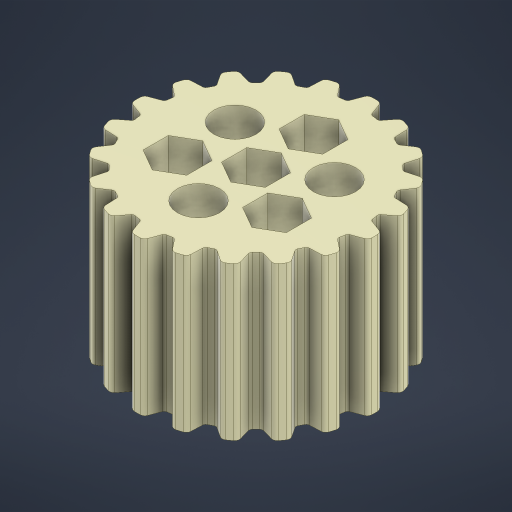
# Autodesk Inventor part: Pulley_Joint2
Saved by Autodesk Inventor 2023 (Build 270158000, 158)
## iProperties
Created: 2023-02-17
Part Number: Pulley_Joint2
Material: ABS Plastic
Document SubType Name: Modeling
Designer: dzw04
Density: 1.06 g/cm^3
Appearance: Smooth - Ash
Author: dzw04
Autodesk Inventor part; units mm, degrees
ref_plane "YZ Plane" through (0, 0, 0) normal (1, 0, 0) x (0, 1, 0)
ref_plane "XZ Plane" through (0, 0, 0) normal (0, 1, 0) x (-1, 0, 0)
ref_plane "XY Plane" through (0, 0, 0) normal (0, 0, 1) x (1, 0, 0)
sketch "Sketch1" plane through (0, 0, 0) normal (0, 1, 0) x (-1, 0, 0)
  arc A0 (-1.7917, 13.431) -> (-2.4464, 13.3273) centre (0, 0) ccw
  arc A1 (-2.8316, 13.4718) -> (-2.4464, 13.3273) centre (-2.5186, 13.7208) ccw
  line L0 (-2.8316, 13.4718) -> (-3.774, 14.6565)
  arc A2 (-3.774, 14.6565) -> (-4.4144, 14.8581) centre (-4.2435, 14.2829) ccw
  arc A3 (-4.4144, 14.8581) -> (-5.162, 14.6152) centre (0, 0) ccw
  arc A4 (-5.162, 14.6152) -> (-5.5616, 14.0756) centre (-4.9622, 14.0494) ccw
  line L1 (-5.5616, 14.0756) -> (-5.6277, 12.5633)
  arc A5 (-5.8545, 12.22) -> (-5.6277, 12.5633) centre (-6.0273, 12.5807) ccw
  arc A6 (-5.8545, 12.22) -> (-6.445, 11.9191) centre (0, 0) ccw
  arc A7 (-6.856, 11.9374) -> (-6.445, 11.9191) centre (-6.6353, 12.2709) ccw
  line L2 (-6.856, 11.9374) -> (-8.1183, 12.7729)
  arc A8 (-8.1183, 12.7729) -> (-8.7898, 12.7668) centre (-8.4495, 12.2726) ccw
  arc A9 (-8.7898, 12.7668) -> (-9.4257, 12.3047) centre (0, 0) ccw
  arc A10 (-9.4257, 12.3047) -> (-9.639, 11.668) centre (-9.0609, 11.8284) ccw
  line L3 (-9.639, 11.668) -> (-9.2345, 10.2093)
  arc A11 (-9.3441, 9.8128) -> (-9.2345, 10.2093) centre (-9.6199, 10.1024) ccw
  arc A12 (-9.3441, 9.8128) -> (-9.8128, 9.3441) centre (0, 0) ccw
  arc A13 (-10.2093, 9.2345) -> (-9.8128, 9.3441) centre (-10.1024, 9.6199) ccw
  line L4 (-10.2093, 9.2345) -> (-11.668, 9.639)
  arc A14 (-11.668, 9.639) -> (-12.3047, 9.4257) centre (-11.8284, 9.0609) ccw
  arc A15 (-12.3047, 9.4257) -> (-12.7668, 8.7898) centre (0, 0) ccw
  arc A16 (-12.7668, 8.7898) -> (-12.7729, 8.1183) centre (-12.2726, 8.4495) ccw
  line L5 (-12.7729, 8.1183) -> (-11.9374, 6.856)
  arc A17 (-11.9191, 6.445) -> (-11.9374, 6.856) centre (-12.2709, 6.6353) ccw
  arc A18 (-11.9191, 6.445) -> (-12.22, 5.8545) centre (0, 0) ccw
  arc A19 (-12.5633, 5.6277) -> (-12.22, 5.8545) centre (-12.5807, 6.0273) ccw
  line L6 (-12.5633, 5.6277) -> (-14.0756, 5.5616)
  arc A20 (-14.0756, 5.5616) -> (-14.6152, 5.162) centre (-14.0494, 4.9622) ccw
  arc A21 (-14.6152, 5.162) -> (-14.8581, 4.4144) centre (0, 0) ccw
  arc A22 (-14.8581, 4.4144) -> (-14.6565, 3.774) centre (-14.2829, 4.2435) ccw
  line L7 (-14.6565, 3.774) -> (-13.4718, 2.8316)
  arc A23 (-13.3273, 2.4464) -> (-13.4718, 2.8316) centre (-13.7208, 2.5186) ccw
  arc A24 (-13.3273, 2.4464) -> (-13.431, 1.7917) centre (0, 0) ccw
  arc A25 (-13.6874, 1.47) -> (-13.431, 1.7917) centre (-13.8275, 1.8446) ccw
  line L8 (-13.6874, 1.47) -> (-15.1053, 0.9398)
  arc A26 (-15.1053, 0.9398) -> (-15.495, 0.393) centre (-14.8952, 0.3778) ccw
  arc A27 (-15.495, 0.393) -> (-15.495, -0.393) centre (0, 0) ccw
  arc A28 (-15.495, -0.393) -> (-15.1053, -0.9398) centre (-14.8952, -0.3778) ccw
  line L9 (-15.1053, -0.9398) -> (-13.6874, -1.47)
  arc A29 (-13.431, -1.7917) -> (-13.6874, -1.47) centre (-13.8275, -1.8446) ccw
  arc A30 (-13.431, -1.7917) -> (-13.3273, -2.4464) centre (0, 0) ccw
  arc A31 (-13.4718, -2.8316) -> (-13.3273, -2.4464) centre (-13.7208, -2.5186) ccw
  line L10 (-13.4718, -2.8316) -> (-14.6565, -3.774)
  arc A32 (-14.6565, -3.774) -> (-14.8581, -4.4144) centre (-14.2829, -4.2435) ccw
  arc A33 (-14.8581, -4.4144) -> (-14.6152, -5.162) centre (0, 0) ccw
  arc A34 (-14.6152, -5.162) -> (-14.0756, -5.5616) centre (-14.0494, -4.9622) ccw
  line L11 (-14.0756, -5.5616) -> (-12.5633, -5.6277)
  arc A35 (-12.22, -5.8545) -> (-12.5633, -5.6277) centre (-12.5807, -6.0273) ccw
  arc A36 (-12.22, -5.8545) -> (-11.9191, -6.445) centre (0, 0) ccw
  arc A37 (-11.9374, -6.856) -> (-11.9191, -6.445) centre (-12.2709, -6.6353) ccw
  line L12 (-11.9374, -6.856) -> (-12.7729, -8.1183)
  arc A38 (-12.7729, -8.1183) -> (-12.7668, -8.7898) centre (-12.2726, -8.4495) ccw
  arc A39 (-12.7668, -8.7898) -> (-12.3047, -9.4257) centre (0, 0) ccw
  arc A40 (-12.3047, -9.4257) -> (-11.668, -9.639) centre (-11.8284, -9.0609) ccw
  line L13 (-11.668, -9.639) -> (-10.2093, -9.2345)
  arc A41 (-9.8128, -9.3441) -> (-10.2093, -9.2345) centre (-10.1024, -9.6199) ccw
  arc A42 (-9.8128, -9.3441) -> (-9.3441, -9.8128) centre (0, 0) ccw
  arc A43 (-9.2345, -10.2093) -> (-9.3441, -9.8128) centre (-9.6199, -10.1024) ccw
  line L14 (-9.2345, -10.2093) -> (-9.639, -11.668)
  arc A44 (-9.639, -11.668) -> (-9.4257, -12.3047) centre (-9.0609, -11.8284) ccw
  arc A45 (-9.4257, -12.3047) -> (-8.7898, -12.7668) centre (0, 0) ccw
  arc A46 (-8.7898, -12.7668) -> (-8.1183, -12.7729) centre (-8.4495, -12.2726) ccw
  line L15 (-8.1183, -12.7729) -> (-6.856, -11.9374)
  arc A47 (-6.445, -11.9191) -> (-6.856, -11.9374) centre (-6.6353, -12.2709) ccw
  arc A48 (-6.445, -11.9191) -> (-5.8545, -12.22) centre (0, 0) ccw
  arc A49 (-5.6277, -12.5633) -> (-5.8545, -12.22) centre (-6.0273, -12.5807) ccw
  line L16 (-5.6277, -12.5633) -> (-5.5616, -14.0756)
  arc A50 (-5.5616, -14.0756) -> (-5.162, -14.6152) centre (-4.9622, -14.0494) ccw
  arc A51 (-5.162, -14.6152) -> (-4.4144, -14.8581) centre (0, 0) ccw
  arc A52 (-4.4144, -14.8581) -> (-3.774, -14.6565) centre (-4.2435, -14.2829) ccw
  line L17 (-3.774, -14.6565) -> (-2.8316, -13.4718)
  arc A53 (-2.4464, -13.3273) -> (-2.8316, -13.4718) centre (-2.5186, -13.7208) ccw
  arc A54 (-2.4464, -13.3273) -> (-1.7917, -13.431) centre (0, 0) ccw
  arc A55 (-1.47, -13.6874) -> (-1.7917, -13.431) centre (-1.8446, -13.8275) ccw
  line L18 (-1.47, -13.6874) -> (-0.9398, -15.1053)
  arc A56 (-0.9398, -15.1053) -> (-0.393, -15.495) centre (-0.3778, -14.8952) ccw
  arc A57 (-0.393, -15.495) -> (0.393, -15.495) centre (0, 0) ccw
  arc A58 (0.393, -15.495) -> (0.9398, -15.1053) centre (0.3778, -14.8952) ccw
  line L19 (0.9398, -15.1053) -> (1.47, -13.6874)
  arc A59 (1.7917, -13.431) -> (1.47, -13.6874) centre (1.8446, -13.8275) ccw
  arc A60 (1.7917, -13.431) -> (2.4464, -13.3273) centre (0, 0) ccw
  arc A61 (2.8316, -13.4718) -> (2.4464, -13.3273) centre (2.5186, -13.7208) ccw
  line L20 (2.8316, -13.4718) -> (3.774, -14.6565)
  arc A62 (3.774, -14.6565) -> (4.4144, -14.8581) centre (4.2435, -14.2829) ccw
  arc A63 (4.4144, -14.8581) -> (5.162, -14.6152) centre (0, 0) ccw
  arc A64 (5.162, -14.6152) -> (5.5616, -14.0756) centre (4.9622, -14.0494) ccw
  line L21 (5.5616, -14.0756) -> (5.6277, -12.5633)
  arc A65 (5.8545, -12.22) -> (5.6277, -12.5633) centre (6.0273, -12.5807) ccw
  arc A66 (5.8545, -12.22) -> (6.445, -11.9191) centre (0, 0) ccw
  arc A67 (6.856, -11.9374) -> (6.445, -11.9191) centre (6.6353, -12.2709) ccw
  line L22 (6.856, -11.9374) -> (8.1183, -12.7729)
  arc A68 (8.1183, -12.7729) -> (8.7898, -12.7668) centre (8.4495, -12.2726) ccw
  arc A69 (8.7898, -12.7668) -> (9.4257, -12.3047) centre (0, 0) ccw
  arc A70 (9.4257, -12.3047) -> (9.639, -11.668) centre (9.0609, -11.8284) ccw
  line L23 (9.639, -11.668) -> (9.2345, -10.2093)
  arc A71 (9.3441, -9.8128) -> (9.2345, -10.2093) centre (9.6199, -10.1024) ccw
  arc A72 (9.3441, -9.8128) -> (9.8128, -9.3441) centre (0, 0) ccw
  arc A73 (10.2093, -9.2345) -> (9.8128, -9.3441) centre (10.1024, -9.6199) ccw
  line L24 (10.2093, -9.2345) -> (11.668, -9.639)
  arc A74 (11.668, -9.639) -> (12.3047, -9.4257) centre (11.8284, -9.0609) ccw
  arc A75 (12.3047, -9.4257) -> (12.7668, -8.7898) centre (0, 0) ccw
  arc A76 (12.7668, -8.7898) -> (12.7729, -8.1183) centre (12.2726, -8.4495) ccw
  line L25 (12.7729, -8.1183) -> (11.9374, -6.856)
  arc A77 (11.9191, -6.445) -> (11.9374, -6.856) centre (12.2709, -6.6353) ccw
  arc A78 (11.9191, -6.445) -> (12.22, -5.8545) centre (0, 0) ccw
  arc A79 (12.5633, -5.6277) -> (12.22, -5.8545) centre (12.5807, -6.0273) ccw
  line L26 (12.5633, -5.6277) -> (14.0756, -5.5616)
  arc A80 (14.0756, -5.5616) -> (14.6152, -5.162) centre (14.0494, -4.9622) ccw
  arc A81 (14.6152, -5.162) -> (14.8581, -4.4144) centre (0, 0) ccw
  arc A82 (14.8581, -4.4144) -> (14.6565, -3.774) centre (14.2829, -4.2435) ccw
  line L27 (14.6565, -3.774) -> (13.4718, -2.8316)
  arc A83 (13.3273, -2.4464) -> (13.4718, -2.8316) centre (13.7208, -2.5186) ccw
  arc A84 (13.3273, -2.4464) -> (13.431, -1.7917) centre (0, 0) ccw
  arc A85 (13.6874, -1.47) -> (13.431, -1.7917) centre (13.8275, -1.8446) ccw
  line L28 (13.6874, -1.47) -> (15.1053, -0.9398)
  arc A86 (15.1053, -0.9398) -> (15.495, -0.393) centre (14.8952, -0.3778) ccw
  arc A87 (15.495, -0.393) -> (15.495, 0.393) centre (0, 0) ccw
  arc A88 (15.495, 0.393) -> (15.1053, 0.9398) centre (14.8952, 0.3778) ccw
  line L29 (15.1053, 0.9398) -> (13.6874, 1.47)
  arc A89 (13.431, 1.7917) -> (13.6874, 1.47) centre (13.8275, 1.8446) ccw
  arc A90 (13.431, 1.7917) -> (13.3273, 2.4464) centre (0, 0) ccw
  arc A91 (13.4718, 2.8316) -> (13.3273, 2.4464) centre (13.7208, 2.5186) ccw
  line L30 (13.4718, 2.8316) -> (14.6565, 3.774)
  arc A92 (14.6565, 3.774) -> (14.8581, 4.4144) centre (14.2829, 4.2435) ccw
  arc A93 (14.8581, 4.4144) -> (14.6152, 5.162) centre (0, 0) ccw
  arc A94 (14.6152, 5.162) -> (14.0756, 5.5616) centre (14.0494, 4.9622) ccw
  line L31 (14.0756, 5.5616) -> (12.5633, 5.6277)
  arc A95 (12.22, 5.8545) -> (12.5633, 5.6277) centre (12.5807, 6.0273) ccw
  arc A96 (12.22, 5.8545) -> (11.9191, 6.445) centre (0, 0) ccw
  arc A97 (11.9374, 6.856) -> (11.9191, 6.445) centre (12.2709, 6.6353) ccw
  line L32 (11.9374, 6.856) -> (12.7729, 8.1183)
  arc A98 (12.7729, 8.1183) -> (12.7668, 8.7898) centre (12.2726, 8.4495) ccw
  arc A99 (12.7668, 8.7898) -> (12.3047, 9.4257) centre (0, 0) ccw
  arc A100 (12.3047, 9.4257) -> (11.668, 9.639) centre (11.8284, 9.0609) ccw
  line L33 (11.668, 9.639) -> (10.2093, 9.2345)
  arc A101 (9.8128, 9.3441) -> (10.2093, 9.2345) centre (10.1024, 9.6199) ccw
  arc A102 (9.8128, 9.3441) -> (9.3441, 9.8128) centre (0, 0) ccw
  arc A103 (9.2345, 10.2093) -> (9.3441, 9.8128) centre (9.6199, 10.1024) ccw
  line L34 (9.2345, 10.2093) -> (9.639, 11.668)
  arc A104 (9.639, 11.668) -> (9.4257, 12.3047) centre (9.0609, 11.8284) ccw
  arc A105 (9.4257, 12.3047) -> (8.7898, 12.7668) centre (0, 0) ccw
  arc A106 (8.7898, 12.7668) -> (8.1183, 12.7729) centre (8.4495, 12.2726) ccw
  line L35 (8.1183, 12.7729) -> (6.856, 11.9374)
  arc A107 (6.445, 11.9191) -> (6.856, 11.9374) centre (6.6353, 12.2709) ccw
  arc A108 (6.445, 11.9191) -> (5.8545, 12.22) centre (0, 0) ccw
  arc A109 (5.6277, 12.5633) -> (5.8545, 12.22) centre (6.0273, 12.5807) ccw
  line L36 (5.6277, 12.5633) -> (5.5616, 14.0756)
  arc A110 (5.5616, 14.0756) -> (5.162, 14.6152) centre (4.9622, 14.0494) ccw
  arc A111 (5.162, 14.6152) -> (4.4144, 14.8581) centre (0, 0) ccw
  arc A112 (4.4144, 14.8581) -> (3.774, 14.6565) centre (4.2435, 14.2829) ccw
  line L37 (3.774, 14.6565) -> (2.8316, 13.4718)
  arc A113 (2.4464, 13.3273) -> (2.8316, 13.4718) centre (2.5186, 13.7208) ccw
  arc A114 (2.4464, 13.3273) -> (1.7917, 13.431) centre (0, 0) ccw
  arc A115 (1.47, 13.6874) -> (1.7917, 13.431) centre (1.8446, 13.8275) ccw
  line L38 (1.47, 13.6874) -> (0.9398, 15.1053)
  arc A116 (0.9398, 15.1053) -> (0.393, 15.495) centre (0.3778, 14.8952) ccw
  arc A117 (0.393, 15.495) -> (-0.393, 15.495) centre (0, 0) ccw
  arc A118 (-0.393, 15.495) -> (-0.9398, 15.1053) centre (-0.3778, 14.8952) ccw
  line L39 (-0.9398, 15.1053) -> (-1.47, 13.6874)
  arc A119 (-1.7917, 13.431) -> (-1.47, 13.6874) centre (-1.8446, 13.8275) ccw
  circle A120 centre (0, 0) radius 17.75
  point P0 (1.47, 13.6874)
  point P1 (0.393, 15.495)
  point P2 (-0.393, 15.495)
  point P3 (-0.9398, 15.1053)
  point P4 (-1.7917, 13.431)
  point P5 (-2.4464, 13.3273)
  point P6 (-2.8316, 13.4718)
  point P7 (-4.4144, 14.8581)
  point P8 (-5.162, 14.6152)
  point P9 (-5.5616, 14.0756)
  point P10 (-5.8545, 12.22)
  point P11 (-6.445, 11.9191)
  point P12 (-8.7898, 12.7668)
  point P13 (-9.4257, 12.3047)
  point P14 (-9.639, 11.668)
  point P15 (-9.3441, 9.8128)
  point P16 (-9.8128, 9.3441)
  point P17 (-10.2093, 9.2345)
  point P18 (-12.3047, 9.4257)
  point P19 (-12.7668, 8.7898)
  point P20 (-11.9191, 6.445)
  point P21 (-12.22, 5.8545)
  point P22 (-12.5633, 5.6277)
  point P23 (-14.6152, 5.162)
  point P24 (-14.8581, 4.4144)
  point P25 (-14.6565, 3.774)
  point P26 (-13.3273, 2.4464)
  point P27 (-13.431, 1.7917)
  point P28 (-13.6874, 1.47)
  point P29 (-15.495, 0.393)
  point P30 (-15.495, -0.393)
  point P31 (-15.1053, -0.9398)
  point P32 (-13.3273, -2.4464)
  point P33 (-13.4718, -2.8316)
  point P34 (-14.8581, -4.4144)
  point P35 (-14.6152, -5.162)
  point P36 (-12.22, -5.8545)
  point P37 (-11.9191, -6.445)
  point P38 (-11.9374, -6.856)
  point P39 (-12.7668, -8.7898)
  point P40 (-12.3047, -9.4257)
  point P41 (-9.8128, -9.3441)
  point P42 (-9.3441, -9.8128)
  point P43 (-9.4257, -12.3047)
  point P44 (-8.7898, -12.7668)
  point P45 (-6.445, -11.9191)
  point P46 (-5.8545, -12.22)
  point P47 (-5.6277, -12.5633)
  point P48 (-5.162, -14.6152)
  point P49 (-4.4144, -14.8581)
  point P50 (-2.4464, -13.3273)
  point P51 (-1.7917, -13.431)
  point P52 (-0.393, -15.495)
  point P53 (0.393, -15.495)
  point P54 (0.9398, -15.1053)
  point P55 (1.7917, -13.431)
  point P56 (2.4464, -13.3273)
  point P57 (2.8316, -13.4718)
  point P58 (4.4144, -14.8581)
  point P59 (5.162, -14.6152)
  point P60 (5.8545, -12.22)
  point P61 (6.445, -11.9191)
  point P62 (8.7898, -12.7668)
  point P63 (9.4257, -12.3047)
  point P64 (9.3441, -9.8128)
  point P65 (9.8128, -9.3441)
  point P66 (10.2093, -9.2345)
  point P67 (12.3047, -9.4257)
  point P68 (12.7668, -8.7898)
  point P69 (12.7729, -8.1183)
  point P70 (12.22, -5.8545)
  point P71 (12.5633, -5.6277)
  point P72 (14.6152, -5.162)
  point P73 (14.8581, -4.4144)
  point P74 (14.6565, -3.774)
  point P75 (13.3273, -2.4464)
  point P76 (13.431, -1.7917)
  point P77 (13.6874, -1.47)
  point P78 (15.495, -0.393)
  point P79 (15.495, 0.393)
  point P80 (15.1053, 0.9398)
  point P81 (13.431, 1.7917)
  point P82 (13.3273, 2.4464)
  point P83 (13.4718, 2.8316)
  point P84 (14.8581, 4.4144)
  point P85 (14.6152, 5.162)
  point P86 (14.0756, 5.5616)
  point P87 (12.22, 5.8545)
  point P88 (11.9191, 6.445)
  point P89 (11.9374, 6.856)
  point P90 (12.7668, 8.7898)
  point P91 (12.3047, 9.4257)
  point P92 (11.668, 9.639)
  point P93 (9.8128, 9.3441)
  point P94 (9.3441, 9.8128)
  point P95 (9.4257, 12.3047)
  point P96 (8.7898, 12.7668)
  point P97 (8.1183, 12.7729)
  point P98 (6.445, 11.9191)
  point P99 (5.8545, 12.22)
  point P100 (5.6277, 12.5633)
  point P101 (5.162, 14.6152)
  point P102 (4.4144, 14.8581)
  point P103 (2.4464, 13.3273)
  point P104 (1.7917, 13.431)
  constraints: 240 point on circle, 121 centre point, 80 end point
extrude "Extrusion1" add sketch "Sketch1" along normal blind 20 contours A119 L39 A118 A117 A116 L38 A115 A114 A113 L37 A112 A111 A110 L36 A109 A108 A107 L35 A106 A105 A104 L34 A103 A102 A101 L33 A100 A99 A98 L32 A97 A96 A95 L31 A94 A93 A92 L30 A91 A90 A89 L29 A88 A87 A86 L28 A85 A84 A83 L27 A82 A81 A80 L26 A79 A78 A77 L25 A76 A75 A74 L24 A73 A72 A71 L23 A70 A69 A68 L22 A67 A66 A65 L21 A64 A63 A62 L20 A61 A60 A59 L19 A58 A57 A56 L18 A55 A54 A53 L17 A52 A51 A50 L16 A49 A48 A47 L15 A46 A45 A44 L14 A43 A42 A41 L13 A40 A39 A38 L12 A37 A36 A35 L11 A34 A33 A32 L10 A31 A30 A29 L9 A28 A27 A26 L8 A25 A24 A23 L7 A22 A21 A20 L6 A19 A18 A17 L5 A16 A15 A14 L4 A13 A12 A11 L3 A10 A9 A8 L2 A7 A6 A5 L1 A4 A3 A2 L0 A1 A0
sketch "Sketch2" plane through (0, 20, 0) normal (0, 1, 0) x (1, 0, 0)
  circle A0 centre (0, 0) radius 7.5 construction
  line L0 (0, 4.2091) -> (-2.85, 5.8546)
  line L1 (-2.85, 5.8546) -> (-2.85, 9.1454)
  line L2 (-2.85, 9.1454) -> (0, 10.7909)
  line L3 (0, 10.7909) -> (2.85, 9.1454)
  line L4 (2.85, 9.1454) -> (2.85, 5.8546)
  line L5 (2.85, 5.8546) -> (0, 4.2091)
  line L6 (0, 3.2909) -> (2.85, 1.6454)
  line L7 (2.85, 1.6454) -> (2.85, -1.6454)
  line L8 (2.85, -1.6454) -> (0, -3.2909)
  line L9 (0, -3.2909) -> (-2.85, -1.6454)
  line L10 (-2.85, -1.6454) -> (-2.85, 1.6454)
  line L11 (-2.85, 1.6454) -> (0, 3.2909)
  circle A1 centre (0, 0) radius 7.5 construction
  line L12 (-3.6452, -2.1046) -> (-3.6452, -5.3954)
  line L13 (-3.6452, -5.3954) -> (-6.4952, -7.0409)
  line L14 (-6.4952, -7.0409) -> (-9.3452, -5.3954)
  line L15 (-9.3452, -5.3954) -> (-9.3452, -2.1046)
  line L16 (-9.3452, -2.1046) -> (-6.4952, -0.4591)
  line L17 (-6.4952, -0.4591) -> (-3.6452, -2.1046)
  circle A2 centre (0, 0) radius 7.5 construction
  line L18 (3.6452, -2.1046) -> (6.4952, -0.4591)
  line L19 (6.4952, -0.4591) -> (9.3452, -2.1046)
  line L20 (9.3452, -2.1046) -> (9.3452, -5.3954)
  line L21 (9.3452, -5.3954) -> (6.4952, -7.0409)
  line L22 (6.4952, -7.0409) -> (3.6452, -5.3954)
  line L23 (3.6452, -5.3954) -> (3.6452, -2.1046)
  point P0 (0, 7.5)
  point P1 (-6.4952, -3.75)
  point P2 (6.4952, -3.75)
  dimension "d2" = 15
  dimension "d3" = 5.7
  dimension "d4" = 5.7
  dimension "d7" = 360
  constraints: 48 end point, 2 coincident, 1 vertical alignment, 80 other
  measures "d3" distance between parallel lines of L7 L10
  measures "d4" distance between parallel lines of L1 L4
extrude "Extrusion2" cut sketch "Sketch2" against normal through all
sketch "Sketch3" plane through (0, 20, 0) normal (0, 1, 0) x (1, 0, 0)
  circle A0 centre (0, 0) radius 7.5
  circle A1 centre (0, -7.5) radius 2.75
  circle A2 centre (6.4952, -3.75) radius 2.75
  circle A3 centre (6.4952, 3.75) radius 2.75
  circle A4 centre (0, 7.5) radius 2.75
  circle A5 centre (-6.4952, 3.75) radius 2.75
  circle A6 centre (-6.4952, -3.75) radius 2.75
  dimension "d11" = 15
  dimension "d12" = 5.5
  dimension "d15" = 360
  constraints: 6 centre point, 1 coincident, 1 vertical alignment, 15 other
  measures "d12" diameter of A1
extrude "Extrusion3" cut sketch "Sketch3" against normal blind 6 contours A3 A0 | A0 A3 | A1 A0 | A0 A1 | A5 A0 | A0 A5
sketch "Sketch4" plane through (0, 0, 0) normal (0, -1, 0) x (1, 0, 0)
  circle A0 centre (0, 0) radius 7.5
  circle A1 centre (0, 7.5) radius 2.75
  circle A2 centre (-6.4952, 3.75) radius 2.75
  circle A3 centre (-6.4952, -3.75) radius 2.75
  circle A4 centre (0, -7.5) radius 2.75
  circle A5 centre (6.4952, -3.75) radius 2.75
  circle A6 centre (6.4952, 3.75) radius 2.75
  dimension "d19" = 15
  dimension "d20" = 5.5
  dimension "d23" = 360
  constraints: 6 centre point, 1 coincident, 1 vertical alignment, 15 other
  measures "d20" diameter of A1
extrude "Extrusion4" cut sketch "Sketch4" against normal blind 6 contours A5 A0 | A0 A5 | A1 A0 | A0 A1 | A3 A0 | A0 A3
body "Solid1"
